potextender (Autodesk Fusion 360 design; units mm, degrees)
Autodesk Fusion 360 part; units mm, degrees
sketch "Sketch1" plane through (0, 0, 0) normal (0, 0, 1) x (1, 0, 0)
  circle A0 centre (0, 0) radius 2.85
  circle A1 centre (0, 0) radius 5
  dimension "d1" = 5.7
  dimension "d2" = 10
  constraint coincident A0.centre A1.centre
  constraint concentric A0 A1
  measures "d1" diameter of A0
  measures "d2" diameter of A1
extrude "Extrude1" add sketch "Sketch1" along normal blind 13 contours A0
ref_plane "WorkPlane1" through (0, 0, -11) normal (0, 0, 1) x (1, 0, 0)
sketch "Sketch2" plane through (0, 0, -11) normal (0, 0, 1) x (1, 0, 0)
  circle A0 centre (0, 0) radius 5
  circle A1 centre (0, 0) radius 3.1
  dimension "d6" = 10
  dimension "d7" = 6.2
  constraint coincident A0.centre A1.centre
  measures "d6" diameter of A0
  measures "d7" diameter of A1
extrude "Extrude2" add sketch "Sketch2" along normal blind 11 contours A0 | A1
extrude "Extrude3" cut sketch "Sketch2" along normal blind 8 contours A1
